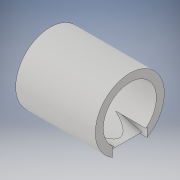
# Autodesk Inventor part: Whistle 3.0
Saved by Autodesk Inventor 2019 (Build 230136000, 136)
## iProperties
Created: 2019-01-22
Part Number: Whistle 3.0
Material: Generic
Document SubType Name: Modeling
Designer: Kepler
Density: 1 g/cm^3
Appearance: Default
Author: Kepler
Autodesk Inventor part; units mm, degrees
ref_plane "YZ Plane" through (0, 0, 0) normal (1, 0, 0) x (0, 1, 0)
ref_plane "XZ Plane" through (0, 0, 0) normal (0, 1, 0) x (-1, 0, 0)
ref_plane "XY Plane" through (0, 0, 0) normal (0, 0, 1) x (1, 0, 0)
ref_plane "Work Plane1" through (0, 0, 10) normal (0, 0, 1) x (1, 0, 0)
sketch "Sketch2" plane through (0, 0, 10) normal (0, 0, 1) x (1, 0, 0)
  line L0 (0, 0) -> (30, 0)
  line L1 (30, 0) -> (30, 3)
  line L2 (30, 3) -> (0, 3)
  line L3 (0, 3) -> (0, 0)
  line L4 (30, 13) -> (0, 13)
  dimension "d11" = 30
  dimension "d12" = 3
  dimension "d13" = 10
  constraints: 10 end point, 3 perpendicular, 2 point on line, 1 horizontal, 1 parallel
  measures "d11" distance of L0.start L0.end
  measures "d12" distance of L0.end L1.end
  measures "d13" distance between parallel lines of L2 L4
revolve "Revolution1" add sketch "Sketch2" angle 360 about axis through (30, 13, 10) along (-1, 0, 0)
sketch "Sketch3" plane through (0, 0, 10) normal (0, 0, 1) x (1, 0, 0)
  line L0 (18.6699, 0) -> (35.6699, 0)
  line L1 (35.6699, 0) -> (35.6699, 5)
  line L2 (35.6699, 5) -> (18.6699, 5)
  line L3 (18.6699, 5) -> (28, 2.5)
  line L4 (28, 2.5) -> (18.6699, 0)
  line L5 (0, 26) -> (0, 0) projected
  line L6 (-3.0148, 0) -> (-5.3111, 0)
  dimension "d17" = 17
  dimension "d19" = 15
  dimension "d20" = 15
  dimension "d21" = 2.5
  dimension "d23" = 28
  dimension "d24" = 5
  dimension "d25" = 5.3111
  dimension "d26" = 7.6699
  constraints: 12 end point, 2 horizontal, 2 perpendicular, 1 collinear, 1 other
  measures "d17" distance of L0.start L0.end
  measures "d19" angle of L3 L2
  measures "d20" angle of L0 L4
  measures "d21" distance from line of L0 L3.end
  measures "d23" distance from line of L5 L3.end
  measures "d24" distance between parallel lines of L0 L2
  measures "d25" distance from line of L6.end L5
  measures "d26" distance from line of L3.end L1
extrude "Extrusion2" cut sketch "Sketch3" along normal mid plane 13
equation "\"d20\" = d19"
body "Solid1"
